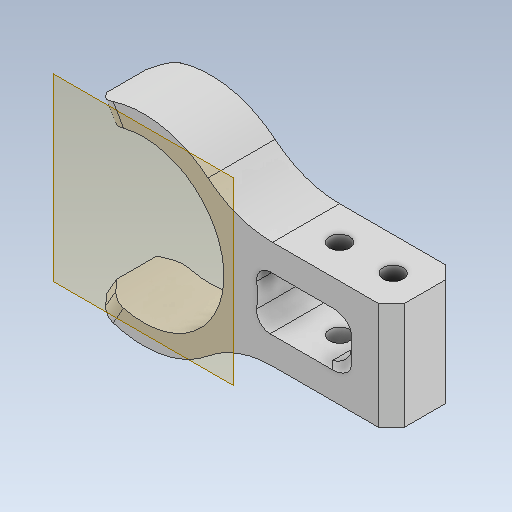
# Autodesk Inventor part: motor_holder_1
Saved by Autodesk Inventor 2020 (Build 240168000, 168)
## iProperties
Created: 2019-06-22
Part Number: motor_holder_1
Material: Generic
Document SubType Name: Modeling
Designer: psrob
Density: 1 g/cm^3
Appearance: Default
Author: psrob
Autodesk Inventor part; units mm, degrees
ref_plane "YZ Plane" through (0, 0, 0) normal (1, 0, 0) x (0, 1, 0)
ref_plane "XZ Plane" through (0, 0, 0) normal (0, 1, 0) x (-1, 0, 0)
ref_plane "XY Plane" through (0, 0, 0) normal (0, 0, 1) x (1, 0, 0)
ref_plane "Work Plane1" through (0, 0, 0) normal (0, 0, 1) x (1, 0, 0)
sketch "Sketch1" plane through (0, 0, 0) normal (0, 0, 1) x (1, 0, 0)
  circle A0 centre (0, 0) radius 12 projected
  circle A1 centre (0, 0) radius 12
  circle A2 centre (0, 0) radius 15
  line L0 (0, 0) -> (0, 15)
  line L1 (0, 0) -> (-7.5, 12.9904)
  line L2 (0, 0) -> (0, -15)
  line L3 (0, 0) -> (-7.5, -12.9904)
  point P0 (-6, 10.3923)
  point P1 (-6, -10.3923)
  dimension "d0" = 24
  dimension "d1" = 30
  dimension "d2" = 30
  dimension "d3" = 30
  constraints: 8 end point, 4 point on circle, 2 centre point, 2 coincident, 1 point on line, 1 vertical
  measures "d0" diameter of A1
  measures "d1" diameter of A2
  measures "d2" angle of L0 L1
  measures "d3" angle of L2 L3
extrude "Extrusion1" add sketch "Sketch1" against normal blind 10 contours A0 L0 A2 L2 | A0 L1 A2 L0 | L2 A2 L3 A0
sketch "Sketch2" plane through (0, 0, 0) normal (0, 0, 1) x (1, 0, 0)
  line L0 (60, -8) -> (20, -8) projected
  line L1 (20, -8) -> (35, -8)
  arc A0 (-7.5, -12.9904) -> (-7.5, 12.9904) centre (0, 0) ccw projected
  line L2 (20, -8) -> (12.6886, -8)
  line L3 (35, -8) -> (35, 8)
  line L4 (35, 8) -> (20, 8)
  line L5 (20, 8) -> (12.6886, 8)
  line L6 (35, -8) -> (35, -4)
  line L7 (35, -4) -> (14.4568, -4)
  line L8 (35, 8) -> (35, 4)
  line L9 (35, 4) -> (14.4568, 4)
  dimension "d6" = 15
  dimension "d7" = 16
  dimension "d8" = 15
  dimension "d9" = 4
  dimension "d10" = 4
  constraints: 18 end point, 4 point on circle, 3 perpendicular, 3 point on line, 2 collinear, 1 vertical
  measures "d6" distance of L0.end L1.end
  measures "d7" distance of L1.end L3.end
  measures "d8" distance of L3.end L4.end
  measures "d9" distance of L1.end L6.end
  measures "d10" distance of L3.end L8.end
extrude "Extrusion2" add sketch "Sketch2" against normal up to surface (10 mm away) contours L0 L2 A0 L7 L3 | L9 A0 L5 L4 L3
fillet "Fillet1" radius 15 2 edges at (12.6886, 8, -5) (12.6886, -8, -5)
thicken "Thicken1" operation add thickness 2 both sides no extend neighbours yes toward (0.9780418, 0.2084088, 0) faces at (14.6706, 3.1261, -6.6667)
fillet "Fillet2" radius 2 2 edges at (16.5227, 4, -5) (16.5227, -4, -5)
thicken "Thicken2" operation add thickness 2 both sides no extend neighbours yes toward (1, 0, 0) faces at (35, -6.6667, -3.3333)
thicken "Thicken3" operation add thickness 2 both sides no extend neighbours yes toward (1, 0, 0) faces at (35, 6.6667, -6.6667)
sketch "Sketch4" plane through (19.2614, -8, -10) normal (0, -1, 0) x (1, 0, 0)
  line L0 (0, 0) -> (0, 10) projected
  line L1 (17.7386, 0) -> (0, 0) projected
  line L2 (17.7386, 10) -> (17.7386, 0) projected
  line L3 (0, 10) -> (17.7386, 10) projected
  line L4 (0, 10) -> (0, 0) projected
  line L5 (0, 5) -> (5, 5)
  line L6 (5, 5) -> (13, 5)
  circle A0 centre (5, 5) radius 1.5
  circle A1 centre (13, 5) radius 1.5
  point P0 (-19.2614, 10)
  dimension "d30" = 5
  dimension "d31" = 8
  dimension "d32" = 3
  dimension "d33" = 3
  constraints: 4 end point, 2 centre point, 2 coincident, 1 horizontal, 1 midpoint, 1 point on line
  measures "d30" distance of L5.start L5.end
  measures "d31" distance of L5.end L6.end
  measures "d32" diameter of A0
  measures "d33" diameter of A1
extrude "Extrusion4" cut sketch "Sketch4" against normal up to surface (16 mm away) contours A0 L6 L5 | L5 L6 A0 | A1
chamfer "Chamfer1" distance 2 angle 45 4 edges at (37, -6, -10) (37, 6, 0) (37, -6, 0) (37, 6, -10)
chamfer "Chamfer2" distance 2 angle 45 4 edges at (-6.75, -11.6913, -10) (-6.75, -11.6913, 0) (-6.75, 11.6913, 0) (-6.75, 11.6913, -10)
fillet "Fillet4" radius 3 4 edges at (-4.9425, -12.5607, -10) (-4.9425, 12.5607, -10) (-4.9425, -12.5607, 0) (-4.9425, 12.5607, 0)
sketch "Sketch5" plane through (18.8944, 4, -10) normal (0, -1, 0) x (1, 0, 0)
  line L0 (16.1056, 10) -> (18.1056, 8) projected
  line L1 (0.3669, 10) -> (16.1056, 10) projected
  line L2 (0.3669, 0) -> (0.3669, 10) projected
  line L3 (16.1056, 0) -> (0.3669, 0) projected
  line L4 (18.1056, 2) -> (16.1056, 0) projected
  line L5 (18.1056, 8) -> (18.1056, 2) projected
  circle A0 centre (5.3669, 5) radius 1.5 projected
  circle A1 centre (13.3669, 5) radius 1.5 projected
  line L6 (0.3669, 10) -> (16.1056, 10) projected
  line L7 (16.1056, 10) -> (10.1056, 10)
  line L8 (10.1056, 10) -> (10.1056, 0)
  point P0 (-18.8944, 10)
  point P1 (10.1056, 10)
  point P2 (10.1056, 0)
  dimension "d43" = 6
  constraints: 4 end point, 1 perpendicular, 1 point on line
  measures "d43" distance of L0.start L7.end
extrude "Extrusion5" add sketch "Sketch5" along normal up to surface (8 mm away) contours L0 L5 L4 L3 L8 L1
chamfer "Chamfer3" distance 2 angle 45 2 edges at (29, 0, -10) (29, 0, 0)
fillet "Fillet5" radius 2 6 edges at (30, -4, -1) (29, -4, -5) (30, -4, -9) (30, 4, -9) (29, 4, -5) (30, 4, -1)
body "Solid1"
